Autodesk Fusion 360 part; units mm, degrees
(part 3 of 3)
  spline S116 degree 3 poles (70.8682, -10.9067) (70.8689, -10.9068) (70.8697, -10.9069) (70.8704, -10.907) (70.9014, -10.9117) (70.8852, -10.9093) (70.8917, -10.9103) (71.1204, -10.9468) (71.4476, -11.0511) (71.5459, -11.0929) (71.549, -11.0943) (71.5519, -11.0955) (71.5545, -11.0966) knots -1.000997 -1.000997 -1.000997 -1.000997 -1.000529 -1.000529 -1.000529 -0.980371 -0.980371 -0.980371 -0.275541 -0.275541 -0.275541 -0.25311 -0.25311 -0.25311 -0.25311
  spline S117 degree 3 poles (71.5545, -11.0966) (71.5904, -11.1173) (71.6451, -11.1483) (71.6906, -11.1738) (73.6297, -12.2612) (75.7255, -12.9133) (77.8404, -13.1384) (81.934, -13.5741) (85.9534, -12.4114) (89.1427, -10.0606) (92.0603, -7.9101) (94.291, -4.7453) (95.2524, -0.9678) knots -0.999138 -0.999138 -0.999138 -0.999138 -0.994208 -0.994208 -0.994208 -0.783863 -0.783863 -0.783863 -0.372519 -0.372519 -0.372519 -0.000783 -0.000783 -0.000783 -0.000783
  line L75 (95.2524, -0.9678) -> (95.2548, -0.9581)
  spline S118 degree 3 poles (95.2548, -0.9581) (95.4077, -0.3591) (95.5351, 0.2728) (95.6121, 1.0629) (95.6881, 1.8436) (95.6857, 2.4844) (95.6857, 2.9324) (95.6857, 2.9387) (95.6857, 2.945) (95.6857, 2.9512) (95.6857, 2.9568) (95.6857, 2.9623) (95.6857, 2.9679) knots -0.993129 -0.993129 -0.993129 -0.993129 -0.542171 -0.542171 -0.542171 0 0 0 0.008156 0.008156 0.008156 0.015382 0.015382 0.015382 0.015382
  spline S119 degree 3 poles (95.6857, 2.9679) (95.6857, 2.9734) (95.6856, 2.979) (95.6856, 2.9845) (95.6855, 2.9908) (95.6855, 2.997) (95.6854, 3.0033) (95.6842, 3.1825) (95.6824, 3.3669) (95.6777, 3.5678) (95.6676, 4.0111) (95.6419, 4.6321) (95.5371, 5.3587) (95.4357, 6.0616) (95.2935, 6.6294) (95.2037, 6.973) (95.2019, 6.98) (95.2001, 6.9869) (95.1983, 6.9939) (95.1966, 7.0001) (95.195, 7.0063) (95.1934, 7.0125) knots -1.0144 -1.0144 -1.0144 -1.0144 -1.007635 -1.007635 -1.007635 -1 -1 -1 -0.809537 -0.809537 -0.809537 -0.396848 -0.396848 -0.396848 0 0 0 0.013642 0.013642 0.013642 0.025729 0.025729 0.025729 0.025729
  spline S120 degree 3 poles (95.1934, 7.0125) (95.1917, 7.0187) (95.1901, 7.0249) (95.1884, 7.031) (95.1865, 7.038) (95.1846, 7.045) (95.1827, 7.0519) (94.9464, 7.9269) (94.6247, 8.8559) (94.1737, 9.8064) (93.7588, 10.6808) (93.2817, 11.4666) (92.7835, 12.1745) (92.5086, 12.5652) (92.2269, 12.9322) (91.9439, 13.2771) (91.8648, 13.3736) (91.7855, 13.4683) (91.7063, 13.5614) (91.6898, 13.5808) (91.6727, 13.6008) (91.6568, 13.6193) knots -1.012984 -1.012984 -1.012984 -1.012984 -1.006884 -1.006884 -1.006884 -1 -1 -1 -0.61483 -0.61483 -0.61483 -0.26383 -0.26383 -0.26383 -0.070103 -0.070103 -0.070103 -0.015926 -0.015926 -0.015926 -0.004648 -0.004648 -0.004648 -0.004648
  spline S121 degree 3 poles (91.6568, 13.6193) (91.6477, 13.6369) (91.6373, 13.6573) (91.6257, 13.6801) knots -0.087703 -0.087703 -0.087703 -0.087703 -0.028603 -0.028603 -0.028603 -0.028603
  spline S122 degree 3 poles (91.6257, 13.6801) (91.6079, 13.7168) (91.585, 13.7666) (91.561, 13.8229) (91.4657, 14.046) (91.2687, 14.6818) (91.1904, 15.0879) (91.1795, 15.1443) (91.1704, 15.1961) (91.1632, 15.2413) knots -0.97664 -0.97664 -0.97664 -0.97664 -0.857358 -0.857358 -0.857358 -0.228377 -0.228377 -0.228377 -0.141153 -0.141153 -0.141153 -0.141153
  spline S123 degree 3 poles (91.1632, 15.2413) (91.1602, 15.3871) (91.1567, 15.5988) (91.1536, 15.8509) (91.1467, 16.4233) (91.1408, 17.2425) (91.1363, 18.2893) (91.1341, 18.7852) (91.1323, 19.3328) (91.1307, 19.9324) knots -0.819896 -0.819896 -0.819896 -0.819896 -0.712378 -0.712378 -0.712378 -0.470371 -0.470371 -0.470371 -0.355745 -0.355745 -0.355745 -0.355745
  spline S124 degree 3 poles (91.1307, 19.9324) (91.1258, 21.7929) (91.1236, 24.153) (91.1236, 27.0233) knots -0.355745 -0.355745 -0.355745 -0.355745 0 0 0 0
  spline S125 degree 3 poles (91.1236, 27.0233) (91.1236, 32.0014) (91.1275, 34.9714) (91.109, 36.9311) (91.0978, 38.1263) (91.0931, 38.9752) (91.0247, 39.8933) (91.002, 40.1983) (90.9719, 40.5054) (90.9337, 40.8147) (90.8313, 41.6439) (90.6842, 42.3291) (90.4598, 43.0655) (90.3687, 43.3647) (90.2864, 43.6042) (90.2412, 43.7314) (90.2331, 43.7542) (90.2265, 43.7726) (90.2223, 43.7843) knots -1 -1 -1 -1 -0.622947 -0.622947 -0.622947 -0.387166 -0.387166 -0.387166 -0.308857 -0.308857 -0.308857 -0.143922 -0.143922 -0.143922 -0.048867 -0.048867 -0.048867 -0.031826 -0.031826 -0.031826 -0.031826
  spline S126 degree 3 poles (90.2223, 43.7843) (90.2122, 43.8145) (90.1952, 43.8645) (90.1814, 43.9046) (89.4663, 45.9843) (88.3746, 47.9244) (86.9378, 49.612) (84.3977, 52.5955) (80.9641, 54.5632) (77.2648, 55.4239) knots -0.999004 -0.999004 -0.999004 -0.999004 -0.992086 -0.992086 -0.992086 -0.63304 -0.63304 -0.63304 -0.001292 -0.001292 -0.001292 -0.001292
  spline S127 degree 3 poles (77.2648, 55.4239) (77.1918, 55.4411) (76.9699, 55.4931) (76.703, 55.5436) (76.1668, 55.6451) (75.7056, 55.6972) (75.2443, 55.7309) (74.6617, 55.7734) (74.1382, 55.7842) (73.4741, 55.7932) (73.4354, 55.7937) (73.3962, 55.7942) (73.3563, 55.7947) (71.868, 55.814) (69.3467, 55.8174) (64.299, 55.8261) knots -0.992248 -0.992248 -0.992248 -0.992248 -0.905652 -0.905652 -0.905652 -0.75 -0.75 -0.75 -0.513738 -0.513738 -0.513738 -0.5 -0.5 -0.5 0 0 0 0
  line L76 (64.299, 55.8261) -> (41.1782, 55.8789)
  line L77 (41.1782, 55.8789) -> (39.8457, 55.8029)
  spline S128 degree 3 poles (40.1314, 50.3146) (40.13, 50.3145) (40.1286, 50.3145) (40.1272, 50.3144) (39.9669, 50.307) (39.8102, 50.2975) (39.6527, 50.2855) (38.9189, 50.2297) (38.0893, 50.062) (37.5809, 49.9247) knots -0.529769 -0.529769 -0.529769 -0.529769 -0.529015 -0.529015 -0.529015 -0.438651 -0.438651 -0.438651 0 0 0 0
  spline S129 degree 3 poles (37.5808, 49.9247) (37.5806, 49.9246) (37.5803, 49.9246) (37.5801, 49.9245) (36.615, 49.665) (35.7195, 49.2885) (34.8796, 48.8197) (33.2356, 47.9019) (31.8242, 46.6784) (30.7274, 45.0372) knots -0.999096 -0.999096 -0.999096 -0.999096 -0.999011 -0.999011 -0.999011 -0.660747 -0.660747 -0.660747 -0.001343 -0.001343 -0.001343 -0.001343
  arc A0 (30.7261, 45.0353) -> (30.7274, 45.0372) centre (30.0622, 45.4817) ccw
  spline S130 degree 3 poles (30.7261, 45.0353) (30.389, 44.5338) (30.0632, 43.9945) (29.7843, 43.4138) (29.4214, 42.6582) (29.16, 41.8653) (28.9586, 41.1056) (28.9585, 41.1053) (28.9584, 41.1051) (28.9584, 41.1048) knots -0.997484 -0.997484 -0.997484 -0.997484 -0.565614 -0.565614 -0.565614 -0.001492 -0.001492 -0.001492 -0.001307 -0.001307 -0.001307 -0.001307
  line L78 (28.9584, 41.1048) -> (28.6512, 39.9559)
  line L79 (28.6512, 39.9559) -> (28.5927, 14.6139)
  line L80 (28.5927, 14.6139) -> (28.5448, 14.3743)
  spline S131 degree 3 poles (28.5448, 14.3743) (28.5175, 14.2369) (28.4997, 14.1528) (28.4763, 14.0452) (28.3765, 13.5859) (28.2654, 13.1616) (28.1463, 12.7744) (27.8705, 11.8778) (27.5477, 11.2066) (27.2669, 10.746) (27.1574, 10.5664) (27.0548, 10.4191) (26.9559, 10.2961) (26.9332, 10.2679) (26.9107, 10.2409) (26.8878, 10.2148) (26.8809, 10.2069) (26.8835, 10.2096) (26.8668, 10.1911) knots -1.000384 -1.000384 -1.000384 -1.000384 -0.950463 -0.950463 -0.950463 -0.737392 -0.737392 -0.737392 -0.247981 -0.247981 -0.247981 -0.057024 -0.057024 -0.057024 -0.013207 -0.013207 -0.013207 0.000075 0.000075 0.000075 0.000075
  spline S132 degree 3 poles (26.8668, 10.1911) (26.8441, 10.1659) (26.7939, 10.1096) (26.7578, 10.0683) (25.8489, 9.0293) (25.1325, 7.8356) (24.6658, 6.5535) (24.2413, 5.3871) (24.0314, 4.1398) (24.0377, 2.8884) (24.0416, 2.1144) (24.1281, 1.339) (24.2968, 0.5808) (24.3773, 0.219) (24.4764, -0.1388) (24.5941, -0.4909) (24.615, -0.5532) (24.6364, -0.6154) (24.6584, -0.6774) (24.6612, -0.6853) (24.664, -0.693) (24.6657, -0.6978) knots -1.000083 -1.000083 -1.000083 -1.000083 -0.98608 -0.98608 -0.98608 -0.633646 -0.633646 -0.633646 -0.31201 -0.31201 -0.31201 -0.113091 -0.113091 -0.113091 -0.018197 -0.018197 -0.018197 -0.001386 -0.001386 -0.001386 0.000763 0.000763 0.000763 0.000763
  spline S133 degree 3 poles (24.6657, -0.6978) (24.678, -0.732) (24.7072, -0.8121) (24.7293, -0.8702) (25.2948, -2.3624) (26.1788, -3.6538) (27.2682, -4.7091) (28.9533, -6.3415) (31.1335, -7.4388) (33.6138, -7.6795) (33.614, -7.6795) (33.6142, -7.6795) (33.6144, -7.6795) knots -1.000544 -1.000544 -1.000544 -1.000544 -0.985474 -0.985474 -0.985474 -0.598384 -0.598384 -0.598384 -0.000479 -0.000479 -0.000479 -0.000441 -0.000441 -0.000441 -0.000441
  spline S134 degree 3 poles (33.6144, -7.6795) (34.1492, -7.7318) (34.6775, -7.742) (35.2011, -7.7151) (36.1495, -7.6664) (37.07, -7.5093) (37.9671, -7.2188) (38.4408, -7.0654) (38.9081, -6.8748) (39.3703, -6.6421) (39.4995, -6.577) (39.6283, -6.5087) (39.7568, -6.4369) (39.8093, -6.4076) (39.8617, -6.3777) (39.914, -6.3472) (39.9199, -6.3438) (39.9228, -6.3421) (39.9258, -6.3403) knots -1 -1 -1 -1 -0.757667 -0.757667 -0.757667 -0.321754 -0.321754 -0.321754 -0.091623 -0.091623 -0.091623 -0.02727 -0.02727 -0.02727 -0.000971 -0.000971 -0.000971 0.001959 0.001959 0.001959 0.001959
  spline S135 degree 3 poles (39.9258, -6.3403) (39.9709, -6.3139) (39.9758, -6.3113) (40.0004, -6.2975) (40.6504, -5.9318) (41.5905, -5.6022) (42.8851, -5.4195) (42.8943, -5.4182) (42.9035, -5.4169) (42.9126, -5.4156) knots -1.001086 -1.001086 -1.001086 -1.001086 -0.965026 -0.965026 -0.965026 -0.011769 -0.011769 -0.011769 -0.004567 -0.004567 -0.004567 -0.004567
  spline S136 degree 3 poles (42.9126, -5.4156) (42.9219, -5.415) (42.9311, -5.4143) (42.9403, -5.4137) (43.0237, -5.4078) (43.1546, -5.4022) (43.4193, -5.395) (43.634, -5.3891) (43.9261, -5.3829) (44.3094, -5.3781) (45.1434, -5.3675) (46.4021, -5.3601) (48.3209, -5.3541) (49.3913, -5.3507) (50.6669, -5.3478) (52.1881, -5.3449) (53.1994, -5.3431) (54.3193, -5.3412) (55.5595, -5.3394) (55.7977, -5.339) (56.0404, -5.3387) (56.2876, -5.3383) knots -0.905937 -0.905937 -0.905937 -0.905937 -0.872881 -0.872881 -0.872881 -0.709686 -0.709686 -0.709686 -0.57731 -0.57731 -0.57731 -0.288645 -0.288645 -0.288645 -0.127612 -0.127612 -0.127612 -0.020552 -0.020552 -0.020552 0.000014 0.000014 0.000014 0.000014
  spline S137 degree 3 poles (56.2876, -5.3383) (57.4962, -5.3362) (58.6063, -5.3344) (59.6274, -5.333) (61.2297, -5.3308) (62.6121, -5.3295) (63.8077, -5.3296) (68.0445, -5.3301) (69.9593, -5.3526) (70.8562, -5.397) (71.221, -5.4151) (71.3919, -5.43) (71.5558, -5.4529) (71.599, -5.459) (71.6397, -5.4651) (71.6824, -5.4717) (71.6859, -5.4722) (71.6881, -5.4725) (71.6937, -5.4734) knots -1.000018 -1.000018 -1.000018 -1.000018 -0.910032 -0.910032 -0.910032 -0.768828 -0.768828 -0.768828 -0.268512 -0.268512 -0.268512 -0.059196 -0.059196 -0.059196 -0.004098 -0.004098 -0.004098 0.000437 0.000437 0.000437 0.000437
  spline S138 degree 3 poles (71.6937, -5.4734) (71.7663, -5.4844) (71.7929, -5.4889) (71.8417, -5.4972) (72.5196, -5.6127) (73.1444, -5.8054) (73.6497, -6.0158) (73.8426, -6.0962) (74.0181, -6.1793) (74.176, -6.2656) (74.2027, -6.2802) (74.2288, -6.2949) (74.2544, -6.3097) (74.258, -6.3117) (74.2617, -6.3138) (74.2685, -6.3178) knots -1.000529 -1.000529 -1.000529 -1.000529 -0.953236 -0.953236 -0.953236 -0.296798 -0.296798 -0.296798 -0.046102 -0.046102 -0.046102 -0.003874 -0.003874 -0.003874 0.002014 0.002014 0.002014 0.002014
  spline S139 degree 3 poles (74.2685, -6.3178) (74.3056, -6.3392) (74.3861, -6.3849) (74.447, -6.4184) (75.7045, -7.1115) (77.07, -7.5297) (78.422, -7.6736) (81.1212, -7.9609) (83.7635, -7.1983) (85.8819, -5.6368) (87.792, -4.229) (89.2925, -2.1098) (89.9281, 0.394) (89.9282, 0.3943) (89.9282, 0.3946) (89.9283, 0.3949) knots -1.000465 -1.000465 -1.000465 -1.000465 -0.990459 -0.990459 -0.990459 -0.783863 -0.783863 -0.783863 -0.372519 -0.372519 -0.372519 -0.000464 -0.000464 -0.000464 -0.000426 -0.000426 -0.000426 -0.000426
  spline S140 degree 3 poles (89.9283, 0.3949) (89.9284, 0.3951) (89.9284, 0.3954) (89.9285, 0.3957) (90.0087, 0.7088) (90.1034, 1.1962) (90.1423, 1.5958) (90.1917, 2.1025) (90.19, 2.4704) (90.19, 2.9324) (90.19, 2.9377) (90.19, 2.9431) (90.19, 2.9484) knots -0.995923 -0.995923 -0.995923 -0.995923 -0.995571 -0.995571 -0.995571 -0.542171 -0.542171 -0.542171 0 0 0 0.006925 0.006925 0.006925 0.006925
  spline S141 degree 3 poles (90.19, 2.9484) (90.19, 2.9537) (90.19, 2.959) (90.1899, 2.9643) (90.1887, 3.1322) (90.1871, 3.2854) (90.1835, 3.4416) (90.1758, 3.7788) (90.1569, 4.1637) (90.0977, 4.5741) (90.0409, 4.9681) (89.9561, 5.3178) (89.8867, 5.5833) (89.8851, 5.5892) (89.8836, 5.5951) (89.882, 5.6011) knots -1.006483 -1.006483 -1.006483 -1.006483 -1 -1 -1 -0.809537 -0.809537 -0.809537 -0.396848 -0.396848 -0.396848 0 0 0 0.011583 0.011583 0.011583 0.011583
  spline S142 degree 3 poles (89.882, 5.6011) (89.8804, 5.607) (89.8788, 5.6129) (89.8772, 5.6188) (89.7154, 6.218) (89.4949, 6.8471) (89.2086, 7.4505) (88.8849, 8.1326) (88.4776, 8.7746) (88.0324, 9.3634) (87.8975, 9.5419) (87.7591, 9.7155) (87.6186, 9.8839) (87.5679, 9.9447) (87.505, 10.0186) (87.4672, 10.0625) knots -1.005845 -1.005845 -1.005845 -1.005845 -1 -1 -1 -0.61483 -0.61483 -0.61483 -0.178392 -0.178392 -0.178392 -0.046071 -0.046071 -0.046071 0.001713 0.001713 0.001713 0.001713
  spline S143 degree 3 poles (87.4672, 10.0625) (87.4279, 10.1079) (87.42, 10.1175) (87.3986, 10.1431) (87.3892, 10.1543) (87.38, 10.1655) (87.3709, 10.1764) (87.1368, 10.461) (86.966, 10.716) (86.7087, 11.2252) (86.7081, 11.2264) (86.7075, 11.2275) (86.7069, 11.2286) knots -1.0017 -1.0017 -1.0017 -1.0017 -0.930298 -0.930298 -0.930298 -0.898949 -0.898949 -0.898949 -0.008653 -0.008653 -0.008653 -0.006595 -0.006595 -0.006595 -0.006595
  spline S144 degree 3 poles (86.7069, 11.2286) (86.7064, 11.2298) (86.7058, 11.2309) (86.7053, 11.232) (86.6391, 11.366) (86.5725, 11.5109) (86.5068, 11.6647) (86.1023, 12.6121) (85.784, 13.8195) (85.6798, 14.7946) (85.6788, 14.8042) (85.6778, 14.8138) (85.6768, 14.8233) knots -0.996214 -0.996214 -0.996214 -0.996214 -0.994911 -0.994911 -0.994911 -0.857358 -0.857358 -0.857358 -0.025015 -0.025015 -0.025015 -0.015796 -0.015796 -0.015796 -0.015796
  spline S145 degree 3 poles (85.6768, 14.8233) (85.6764, 14.8329) (85.6761, 14.8425) (85.6758, 14.8521) (85.6707, 14.9989) (85.6639, 15.3283) (85.6584, 15.7846) (85.6511, 16.382) (85.6452, 17.2106) (85.6407, 18.2655) (85.6385, 18.7652) (85.6366, 19.3158) (85.635, 19.9179) knots -0.910204 -0.910204 -0.910204 -0.910204 -0.896967 -0.896967 -0.896967 -0.712378 -0.712378 -0.712378 -0.470371 -0.470371 -0.470371 -0.355745 -0.355745 -0.355745 -0.355745
  spline S146 degree 3 poles (85.635, 19.9179) (85.6301, 21.7863) (85.6279, 24.1502) (85.6279, 27.0233) knots -0.355745 -0.355745 -0.355745 -0.355745 0 0 0 0
  spline S147 degree 3 poles (85.6279, 27.0233) (85.6279, 32.0041) (85.6315, 34.9805) (85.6136, 36.8794) (85.5986, 38.4681) (85.5891, 39.2533) (85.4794, 40.1414) (85.4256, 40.5775) (85.3049, 41.1286) (85.2027, 41.4641) (85.127, 41.7123) (85.0816, 41.8385) (85.0488, 41.9304) (85.0383, 41.9596) (85.0316, 41.9776) (85.0176, 42.0197) knots -1 -1 -1 -1 -0.622947 -0.622947 -0.622947 -0.308857 -0.308857 -0.308857 -0.143922 -0.143922 -0.143922 -0.034026 -0.034026 -0.034026 0.000931 0.000931 0.000931 0.000931
  spline S148 degree 3 poles (85.0176, 42.0197) (85.0031, 42.0631) (84.9734, 42.1501) (84.9502, 42.2157) (84.4537, 43.6212) (83.7075, 44.9286) (82.7533, 46.0494) (81.0363, 48.0661) (78.6335, 49.4641) (76.0143, 50.0724) (76.0139, 50.0725) (76.0135, 50.0726) (76.0131, 50.0726) knots -1.0003 -1.0003 -1.0003 -1.0003 -0.983934 -0.983934 -0.983934 -0.63304 -0.63304 -0.63304 -0.000881 -0.000881 -0.000881 -0.000793 -0.000793 -0.000793 -0.000793
  spline S149 degree 3 poles (76.0131, 50.0726) (76.0127, 50.0727) (76.0124, 50.0728) (76.012, 50.0729) (75.9459, 50.0885) (75.8316, 50.1153) (75.6814, 50.1438) (75.4289, 50.1915) (75.1047, 50.2308) (74.8445, 50.2498) (74.4054, 50.2818) (73.9953, 50.2903) (73.2853, 50.2995) (71.8713, 50.3178) (69.3376, 50.3217) (64.2895, 50.3304) (64.2895, 50.3304) (64.2894, 50.3304) (64.2893, 50.3304) knots -0.995394 -0.995394 -0.995394 -0.995394 -0.994872 -0.994872 -0.994872 -0.905652 -0.905652 -0.905652 -0.75 -0.75 -0.75 -0.5 -0.5 -0.5 0 0 0 0.000007 0.000007 0.000007 0.000007
  line L81 (64.2893, 50.3304) -> (41.3286, 50.3829)
  line L82 (41.3286, 50.3829) -> (40.1314, 50.3146)
  dimension "d21" = 4.6957
  dimension "d22" = -0.8
sketch "Sketch8" plane through (48.0053, 0, 0) normal (1, 0, 0) x (0, 1, 0)
  line L0 (-5, -0.8549) -> (-12, -0.8549)
  line L1 (-12, -0.8549) -> (-12, -5.3551)
  line L2 (-12, -5.3551) -> (-5, -5.3551)
  line L3 (-5, -5.3551) -> (-5, -0.8549)
  line L4 (-12, -6.1) -> (-12, -10.6)
  line L5 (-12, -10.6) -> (-3, -6.1)
  line L6 (-3, -6.1) -> (-12, -6.1)
  dimension "d23" = 4.5
  dimension "d24" = 9
  constraint vertical L4
  constraint perpendicular L4 L6
  measures "d23" distance of L4.start L4.end
  measures "d24" distance of L4.start L5.end
extrude "Extrude4" add sketch "Sketch6" against normal blind 5 separate body contours S89 S90 A0 | S106 S107 S108 L72 L73 S109 S110 S111 S112 S113 S114 S115 L74 S116 S117 L75 S118 S119 S120 S121 S122 S123 S124 S125 S126 S127 L76 L77 picked at (29.7441, 45.0553) makes body 4
extrude "Extrude5" cut 1 faces at (81.4228, 0, 2.7268) along direction (0, -1, 0) blind 2 on bodies 2 bodies 2
combine "Combine1" operation add target body 4 tool bodies 2
equation "d8 = d7"
equation "d9 = d7"
equation "d10 = d7"
equation "d11 = d9"
equation "d12 = d9"
equation "d13 = d11"
equation "d14 = d13"
equation "d15 = d14"
